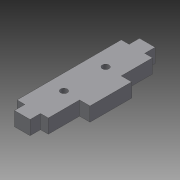
# Autodesk Inventor part: Frame_Lower_Vertical_Plate_B
Saved by Autodesk Inventor 2014 (Build 180170000, 170)
## iProperties
Created: 2014-08-27
Part Number: Frame_Lower_Vertical_Plate_B
Material: Generic
Document SubType Name: Modeling
Designer: ThatOtherGuy
Density: 1 g/cm^3
Appearance: Default
Author: ThatOtherGuy
Autodesk Inventor part; units mm, degrees
ref_plane "YZ Plane" through (0, 0, 0) normal (1, 0, 0) x (0, 1, 0)
ref_plane "XZ Plane" through (0, 0, 0) normal (0, 1, 0) x (-1, 0, 0)
ref_plane "XY Plane" through (0, 0, 0) normal (0, 0, 1) x (1, 0, 0)
sketch "Sketch1" plane through (0, 0, 0) normal (0, 0, 1) x (1, 0, 0)
  line L0 (0, 0) -> (3.75, 0)
  line L1 (3.75, 0) -> (3.75, -5)
  line L2 (3.75, -5) -> (11.25, -5)
  line L3 (11.25, -5) -> (11.25, 0)
  line L4 (11.25, 0) -> (15, 0)
  line L5 (15, 0) -> (15, 15)
  line L6 (15, 15) -> (20, 15)
  line L7 (20, 15) -> (20, 35)
  line L8 (20, 35) -> (15, 35)
  line L9 (15, 35) -> (15, 50)
  line L10 (15, 50) -> (11.25, 50)
  line L11 (11.25, 50) -> (11.25, 55)
  line L12 (11.25, 55) -> (3.75, 55)
  line L13 (3.75, 55) -> (3.75, 50)
  line L14 (3.75, 50) -> (0, 50)
  line L15 (0, 50) -> (0, 0)
  circle A0 centre (7.5, 35) radius 1.6
  circle A1 centre (7.5, 15) radius 1.6
  line L16 (7.5, 15) -> (7.5, 35)
  point P0 (20, 25)
  point P1 (0, 25)
  point P2 (7.5, -5)
  point P3 (7.5, 25)
  dimension "d0" = 5
  dimension "d1" = 50
  dimension "d2" = 20
  dimension "d3" = 7.5
  dimension "d4" = 15
  dimension "d5" = 3.2
  dimension "d6" = 20
  constraints: 34 end point, 12 parallel, 8 equal length, 4 midpoint, 3 perpendicular, 2 centre point, 2 horizontal alignment, 2 vertical alignment, 1 collinear, 1 equal radius, 1 horizontal
  measures "d0" distance of L12.end L13.end
  measures "d1" distance of L14.end L0.start
  measures "d2" distance of L6.end L7.end
  measures "d3" distance of L11.end L12.end
  measures "d4" distance between parallel lines of L15 L9
  measures "d5" diameter of A1
  measures "d6" distance of L16.start L16.end
extrude "Extrusion1" add sketch "Sketch1" along normal blind 6.731
equation "\"d7\" = THICKB"
equation "\"THICKA\" = 3.175"
equation "\"THICKB\" = 6.731"
equation "\"THICKC\" = 12.7"
equation "\"BALLDIA\" = 12"
equation "\"MAGDIA\" = 9.5"
equation "\"THICKPLY\" = 5"
body "Solid1"
